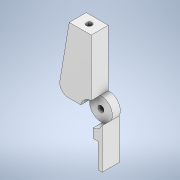
# Autodesk Inventor part: pliers
Saved by Autodesk Inventor 2020 (Build 240168000, 168)
## iProperties
Created: 2019-12-24
Part Number: pliers
Material: ABS Plastic
Document SubType Name: Modeling
Designer: metal
Density: 1.06 g/cm^3
Appearance: Smooth - White
Author: metal
Autodesk Inventor part; units mm, degrees
ref_plane "YZ Plane" through (0, 0, 0) normal (1, 0, 0) x (0, 1, 0)
ref_plane "XZ Plane" through (0, 0, 0) normal (0, 1, 0) x (-1, 0, 0)
ref_plane "XY Plane" through (0, 0, 0) normal (0, 0, 1) x (1, 0, 0)
sketch "Sketch1" plane through (0, 0, 0) normal (0, 0, 1) x (1, 0, 0)
  circle A0 centre (0, 0) radius 4
  line L0 (0, 24) -> (-8, 24)
  line L1 (0, 24) -> (0, 4)
  line L2 (-11.904343, 0.869542) -> (-3.904343, 0.869542)
  line L3 (-11.904343, 0.869542) -> (-8, 24)
  dimension "d0" = 8
  dimension "d6" = 8
  dimension "d94" = 20
  dimension "d95" = 8
  constraints: 8 end point, 2 horizontal, 2 point on circle, 1 centre point, 1 coincident, 1 vertical
  measures "d0" diameter of A0
  measures "d6" distance of L0.start L0.end
  measures "d94" distance of L0.start L1.end
  measures "d95" distance of L2.start L2.end
extrude "Extrusion1" add sketch "Sketch1" along normal mid plane 6
sketch "Sketch2" plane through (0, 0, 3) normal (0, 0, 1) x (1, 0, 0)
  circle A0 centre (0, 0) radius 4
  constraints: 1 centre point, 1 coincident
extrude "Extrusion2" cut sketch "Sketch2" against normal blind 3.2
sketch "Sketch4" plane through (-8, 24, 3) normal (0, 1, 0) x (1, 0, 0)
  line L0 (8, 6) -> (8, 0) projected
  line L1 (0, 0) -> (8, 6)
  line L2 (8, 0) -> (0, 0) projected
  line L3 (0, 6) -> (0, 0) projected
  line L4 (8, 0) -> (0, 6)
  circle A0 centre (4, 3) radius 1
  line L5 (3.2, 2.4) -> (3.2, 3.6)
  point P0 (8, 3)
  dimension "d17" = 2
  dimension "d93" = 1.2
  constraints: 6 end point, 2 point on circle, 1 centre point, 1 midpoint, 1 vertical
  measures "d17" diameter of A0
  measures "d93" distance of L5.start L5.end
extrude "Extrusion4" cut sketch "Sketch4" against normal blind 5 contours A0 L4 L1 | L1 L4 A0 | A0 L1 L4 | L1 L5 L4
sketch "Sketch8" plane through (0, 0, -0.2) normal (0, 0, 1) x (1, 0, 0)
  arc A0 (-3.904343, 0.869542) -> (0, 4) centre (0, 0) ccw
  constraints: 1 coincident
hole "Hole3" at (0, 0, -0.2) direction (0, 0, -1) diameter 2.1 end through all
sketch "Sketch9" plane through (0, 0, 0) normal (0, 0, 1) x (1, 0, 0)
  line L0 (0, 4) -> (0, 24) construction
  line L1 (0, 24) -> (-8, 24) construction
  line L2 (-3.267949, 22.732051) -> (-9.312105, 0.174954) construction
  line L3 (-11.904343, 0.869542) -> (-3.904343, 0.869542) construction
  arc A0 (0, 4) -> (-3.904343, 0.869542) centre (0, 0) ccw construction
  arc A1 (-3.904343, 0.869542) -> (0, 4) centre (0, 0) ccw
  line L4 (0, 31.995011) -> (0, -23.970063) construction
  arc A2 (-3.904343, 0.869542) -> (0, 4) centre (0, 0) ccw construction
  line L5 (0.446045, -3.975053) -> (0.446045, -10.975053)
  line L6 (3.846045, -1.099061) -> (3.846045, -15.975053)
  line L7 (0.446045, -10.975053) -> (2.246045, -10.975053)
  line L8 (2.246045, -10.975053) -> (2.246045, -15.975053)
  line L9 (2.246045, -15.975053) -> (3.846045, -15.975053)
  point P0 (0.446045, -3.975053)
  dimension "d90" = 7
  dimension "d91" = 3.4
  dimension "d92" = 1.8
  constraints: 10 end point, 2 perpendicular, 2 point on circle, 2 vertical, 1 horizontal
  measures "d90" distance of L5.start L5.end
  measures "d91" horizontal distance of L6.start L5.start
  measures "d92" distance of L5.end L7.end
extrude "Extrusion5" add sketch "Sketch9" along normal mid plane 6
sketch "Sketch10" plane through (0, 0, -3) normal (0, 0, -1) x (-1, 0, 0)
  circle A0 centre (0, 0) radius 1.05 projected
  circle A1 centre (0, 0) radius 1.8
  dimension "d62" = 3.6
  constraints: 1 centre point, 1 coincident
  measures "d62" diameter of A1
extrude "Extrusion6" cut sketch "Sketch10" against normal blind 1
fillet "Fillet2" radius 3 1 edges at (-11.9043, 0.8695, 0)
sketch "Sketch17" plane through (0, 0, 0) normal (0, 0, 1) x (1, 0, 0)
  line L0 (-11.313669, 4.368869) -> (-8, 24)
  line L1 (-8.238136, 22.589215) -> (-8.238136, 19.389215)
  line L2 (-8.238136, 19.389215) -> (-8.778285, 19.389215)
  point P0 (0, 0)
  dimension "d107" = 3.2
  constraints: 4 end point, 2 point on line, 1 horizontal, 1 vertical
  measures "d107" distance of L1.start L1.end
extrude "Extrusion10" cut sketch "Sketch17" along normal mid plane 4
sketch "Sketch18" plane through (-8.238136, 19.389215, -2) normal (-1, 0, 0) x (0, 0, 1)
  line L0 (0, 3.2) -> (4, 3.2) projected
  line L1 (0, 3.2) -> (0, 0) projected
  point P0 (2, -19.389215)
  point P1 (2, 1.6)
  dimension "d110" = 1.6
  dimension "d111" = 2
  measures "d110" distance from line of L0 point (2, 1.6)
  measures "d111" distance from line of L1 point (2, 1.6)
hole "Hole5" at (-8.238136, 20.989215, 0) direction (1, 0, 0) diameter 0.8 depth 4 tip angle 118
move faces "Move1" translate (-0.25, 0, 0) faces at (3.846045, -11.016389, -0.066667)
move faces "Move2" translate (-0.25, 0, 0) faces at (0, 17.333333, -0.066667)
move faces "Move3" translate (0, 3.75, 0) faces at (1.646045, -10.975053, 1)
body "Solid1"
